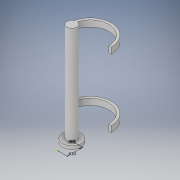
# Autodesk Inventor part: pincherleft
Saved by Autodesk Inventor 2017 (Build 210142000, 142)
## iProperties
Created: 2017-11-18
Part Number: pincherleft
Material: Generic
Document SubType Name: Modeling
Designer: User
Density: 1 g/cm^3
Appearance: Default
Author: User
Autodesk Inventor part; units mm, degrees
ref_plane "YZ Plane" through (0, 0, 0) normal (1, 0, 0) x (0, 1, 0)
ref_plane "XZ Plane" through (0, 0, 0) normal (0, 1, 0) x (-1, 0, 0)
ref_plane "XY Plane" through (0, 0, 0) normal (0, 0, 1) x (1, 0, 0)
sketch "Sketch1" plane through (0, 0, 0) normal (0, 1, 0) x (-1, 0, 0)
  circle A0 centre (0, 0) radius 5.08
  dimension "d0" = 10.16
  constraints: 1 centre point, 1 coincident
  measures "d0" diameter of A0
extrude "Extrusion1" add sketch "Sketch1" along normal blind 101.6
sketch "Sketch2" plane through (0, 101.6, 0) normal (0, 1, 0) x (1, 0, 0)
  circle A0 centre (0, 0) radius 5.08 projected
  line L0 (0, 0) -> (-2.54, 0)
  line L1 (38.1, 0) -> (40.64, 0)
  arc A1 (38.1, 0) -> (0, 0) centre (19.05, 0) ccw
  arc A2 (40.64, 0) -> (-2.54, 0) centre (19.05, 0) ccw
  line L2 (38.1, 0) -> (40.64, 0) construction
  line L3 (5.08, 0) -> (-2.54, 0) construction
  line L4 (-2.54, 0) -> (5.08, 0)
  line L5 (38.1, 0) -> (40.64, 0)
  dimension "d64" = 2.54
  dimension "d65" = 2.54
  dimension "d66" = 38.1
  dimension "d67" = 19.05
  dimension "d68" = 180
  dimension "d69" = 21.59
  constraints: 12 end point, 4 point on circle, 2 centre point, 2 coincident, 2 horizontal, 1 horizontal alignment, 1 other
  measures "d64" distance of L0.start L0.end
  measures "d65" distance of L1.start L1.end
  measures "d66" distance of L1.start L0.start
  measures "d67" distance of L1.start point (19.05, 0)
  measures "d68" angle of L3 L2
  measures "d69" distance of A2.centre L1.end
ref_plane "Work Plane2" through (0, 31.75, 0) normal (0, 1, 0) x (1, 0, 0)
sketch "Sketch3" plane through (0, 31.75, 0) normal (0, 1, 0) x (1, 0, 0)
  line L0 (0, 0) -> (-2.54, 0)
  line L1 (38.1, 0) -> (40.64, 0)
  arc A0 (38.1, 0) -> (0.6773, 5.0346) centre (19.05, 0) ccw
  line L2 (5.08, 0) -> (0, 0) construction
  arc A1 (40.64, 0) -> (-2.032, 4.6559) centre (19.05, 0) ccw
  line L3 (5.08, 0) -> (-3.81, 0) construction
  line L4 (38.1, 0) -> (40.64, 0) construction
  circle A2 centre (0, 0) radius 5.08 projected
  arc A3 (40.64, 0) -> (-2.032, 4.6559) centre (19.05, 0) ccw
  arc A4 (38.1, 0) -> (0.6773, 5.0346) centre (19.05, 0) ccw
  arc A5 (0.6773, 5.0346) -> (-2.032, 4.6559) centre (0.1812, -1.2959) ccw
  line L5 (40.64, 0) -> (38.1, 0)
  line L6 (5.08, 0) -> (-2.921, 0)
  point P0 (1.5835, 6.1394)
  dimension "d48" = 2.54
  dimension "d49" = 2.54
  dimension "d50" = 38.1
  dimension "d51" = 19.05
  dimension "d53" = 180
  dimension "d55" = 6.35
  constraints: 14 end point, 14 point on circle, 5 centre point, 2 coincident, 2 concentric, 2 horizontal, 1 point on line, 3 other
  measures "d48" distance of L0.start L0.end
  measures "d49" distance of L1.start L1.end
  measures "d50" distance of L1.start L0.start
  measures "d51" distance of L1.start point (19.05, 0)
  measures "d53" angle of L3 L4
  measures "d55" radius of A5
extrude "Extrusion4" add sketch "Sketch3" against normal blind 6.35 contours A0 A2 A1 L1 | A5 A2 picked at (-0.5473, 5.0202)
extrude "Extrusion5" add sketch "Sketch2" against normal blind 6.35 contours A1 L0 A2 A0 | A0 A2 L1 A1
sketch "Sketch4" plane through (0, 0, 0) normal (0, -1, 0) x (1, 0, 0)
  circle A0 centre (0, 0) radius 9.525
  dimension "d72" = 19.05
  constraints: 1 centre point, 1 coincident
  measures "d72" diameter of A0
extrude "Extrusion6" add sketch "Sketch4" along normal blind 3.175
sketch "Sketch5" plane through (0, -3.175, 0) normal (0, -1, 0) x (1, 0, 0)
  point P0 (0, 0)
  point P1 (0, 15.2083)
  point P2 (0, -0.7937)
  point P3 (0.7937, 0)
  point P4 (-0.7937, 0)
  dimension "d75" = 1.5875
  dimension "d76" = 16.002
  dimension "d77" = 0.7937
  dimension "d78" = 0.7937
  measures "d75" distance of point (-0.794, 0) point (0.794, 0)
  measures "d76" distance of point (0, 15.208) point (0, -0.794)
  measures "d77" distance of point (0, 0) point (0, -0.794)
  measures "d78" distance of point (0, 0) point (0.794, 0)
equation "\"d67\" = 0.5 * d66"
equation "\"d51\" = 0.5 * d50"
body "Solid1"
